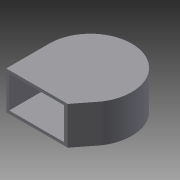
# Autodesk Inventor part: FanRadial40mm
Saved by Autodesk Inventor 2015 (Build 190159000, 159)
## iProperties
Created: 2014-12-06
Part Number: FanRadial40mm
Material: Generic
Document SubType Name: Modeling
Designer: Jack
Density: 1 g/cm^3
Appearance: Default
Author: Jack
Autodesk Inventor part; units mm, degrees
ref_plane "YZ Plane" through (0, 0, 0) normal (1, 0, 0) x (0, 1, 0)
ref_plane "XZ Plane" through (0, 0, 0) normal (0, 1, 0) x (-1, 0, 0)
ref_plane "XY Plane" through (0, 0, 0) normal (0, 0, 1) x (1, 0, 0)
sketch "Sketch1" plane through (0, 0, 0) normal (0, 0, 1) x (1, 0, 0)
  line L0 (0, 0) -> (123.3934, 0) construction
  line L1 (123.3934, 0) -> (123.3934, -69.4088) construction
  line L2 (123.3934, -69.4088) -> (0, -69.4088) construction
  line L3 (0, -69.4088) -> (0, 0) construction
  line L4 (36.4003, -60.1) -> (67.6003, -60.1)
  line L5 (67.6003, -60.1) -> (75.0895, -50.4798)
  line L6 (36.4003, -60.1) -> (36.4003, -37.8811)
  arc A0 (57.111, -17.4004) -> (36.4003, -37.8811) centre (57.2471, -38.25) ccw
  arc A1 (75.0895, -50.4798) -> (57.111, -17.4004) centre (57.2503, -38.75) ccw
  dimension "d8" = 21.35
  dimension "d11" = 20.85
  dimension "d12" = 20.85
  dimension "d13" = 21.35
  dimension "d14" = 127.9
  dimension "d15" = 57.2503
  dimension "d16" = 0.5
  dimension "d18" = 38.25
  dimension "d21" = 31.2
  constraints: 8 end point, 4 point on circle, 2 centre point, 2 horizontal, 1 tangent, 1 vertical, 2 other
  measures "d8" radius of A1
  measures "d11" radius of A0
  measures "d12" distance from line of A1.centre L6
  measures "d13" distance from line of A1.centre L4
  measures "d14" angle of L5 L4
  measures "d15" horizontal distance of point (0, 0) A1.centre
  measures "d16" distance of A0.centre A1.centre
  measures "d18" vertical distance of point (0, 0) A0.centre
  measures "d21" distance of L4.start L4.end
extrude "Extrusion1" add sketch "Sketch1" along normal blind 19.2
shell "Shell1" thickness 1.5 removed faces 0
sketch "Sketch2" plane through (36.4003, -60.1, 0) normal (0, -1, 0) x (1, 0, 0)
  line L0 (1.5, 17.7) -> (30.4668, 17.7) projected
  line L1 (1.5, 1.5) -> (1.5, 17.7) projected
  line L2 (30.4668, 1.5) -> (30.4668, 17.7) projected
  line L3 (1.5, 1.5) -> (30.4668, 1.5) projected
  point P0 (-36.4003, 0)
extrude "Extrusion2" cut sketch "Sketch2" against normal blind 2
sketch "Sketch3" plane through (37.9003, -60.1, 1.5) normal (0, 0, 1) x (1, 0, 0)
  line L0 (28.9668, 1.5) -> (35.968, 10.4935) projected
  line L1 (28.9668, 0) -> (0, 0) projected
  line L2 (28.9668, 0) -> (28.9668, 1.5) projected
  line L3 (28.9668, 1.5) -> (27.7991, 0)
  point P0 (-37.9003, 60.1)
  constraints: 2 end point, 1 collinear, 1 point on line
extrude "Extrusion3" add sketch "Sketch3" along normal up to next
body "Solid1"
